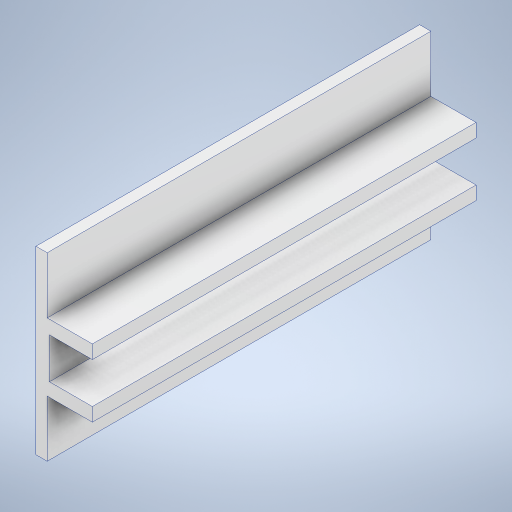
# Autodesk Inventor part: MainRails
Saved by Autodesk Inventor 2024 (Build 280153000, 153)
## iProperties
Created: 2023-08-20
Part Number: MainRails
Material: Aluminum 6061
Document SubType Name: Modeling
Designer: KirikDK
Mass: 4130.47 g
Surface Area: 1743.17 cm^2
Volume: 1529.8 cm^3
Density: 2.7 g/cm^3
Appearance: Aluminum - Flat
Author: KirikDK
Autodesk Inventor part; units mm, degrees
ref_plane "YZ Plane" through (0, 0, 0) normal (1, 0, 0) x (0, 1, 0)
ref_plane "XZ Plane" through (0, 0, 0) normal (0, 1, 0) x (-1, 0, 0)
ref_plane "XY Plane" through (0, 0, 0) normal (0, 0, 1) x (1, 0, 0)
sketch "Sketch1" plane through (0, 0, 0) normal (0, 1, 0) x (-1, 0, 0)
  line L0 (0, 279.3478) -> (-39.1304, 279.3478)
  line L1 (-39.1304, 279.3478) -> (-39.1304, -195.6522)
  line L2 (-39.1304, -195.6522) -> (0, -195.6522)
  line L3 (0, -195.6522) -> (0, 279.3478)
  line L4 (-39.1304, 279.3478) -> (-29.1304, 279.3478)
  line L5 (-29.1304, 254.3478) -> (-39.1304, 254.3478)
  line L6 (-39.1304, 254.3478) -> (-39.1304, 279.3478)
  line L7 (-39.1304, -195.6522) -> (-29.1304, -195.6522)
  line L8 (-29.1304, -170.6522) -> (-39.1304, -170.6522)
  line L9 (-39.1304, -170.6522) -> (-39.1304, -195.6522)
  point P0 (0, 0)
  point P1 (-39.1304, 254.3478)
  dimension "d0" = 475
  dimension "d4" = 25
  dimension "d5" = 25
  constraints: 20 end point, 4 parallel, 3 horizontal, 1 perpendicular
  measures "d0" distance of L2.end L0.start
  measures "d4" distance between parallel lines of L0 L5
  measures "d5" distance between parallel lines of L2 L8
extrude "Extrusion1" add sketch "Sketch1" along normal blind 160
sketch "Sketch2" plane through (0, 0, 279.3478) normal (0, 0, 1) x (1, 0, 0)
  line L0 (0, 160) -> (39.1304, 160) projected
  line L1 (0, 160) -> (39.1304, 160)
  line L2 (39.1304, 160) -> (39.1304, 0)
  line L3 (39.1304, 0) -> (0, 0)
  line L4 (0, 0) -> (0, 160)
  line L5 (39.1304, 160) -> (29.1304, 160)
  line L6 (29.1304, 160) -> (29.1304, 110)
  line L7 (29.1304, 110) -> (39.1304, 110)
  line L8 (39.1304, 110) -> (39.1304, 160)
  line L9 (39.1304, 0) -> (29.1304, 0)
  line L10 (29.1304, 0) -> (29.1304, 50)
  line L11 (29.1304, 50) -> (39.1304, 50)
  line L12 (39.1304, 50) -> (39.1304, 0)
  circle A0 centre (39.1304, 80) radius 18
  line L13 (31.1304, 75) -> (39.1304, 75)
  line L14 (39.1304, 75) -> (39.1304, 98)
  line L15 (39.1304, 98) -> (31.1304, 98)
  line L16 (31.1304, 98) -> (31.1304, 75)
  line L17 (31.1304, 75) -> (39.1304, 75)
  line L18 (39.1304, 75) -> (39.1304, 62)
  line L19 (39.1304, 62) -> (31.1304, 62)
  line L20 (31.1304, 62) -> (31.1304, 75)
  line L21 (39.1304, 0) -> (39.1304, 160) projected
  line L22 (0, 160) -> (19.1304, 160)
  line L23 (19.1304, 160) -> (19.1304, 0)
  line L24 (19.1304, 0) -> (0, 0)
  line L25 (0, 0) -> (0, 160)
  point P0 (0, 0)
  point P1 (34.1304, 110)
  point P2 (34.1304, 160)
  point P3 (39.1304, 50)
  point P4 (39.1304, 110)
  dimension "d6" = 10
  dimension "d7" = 50
  dimension "d8" = 50
  dimension "d9" = 8
  dimension "d10" = 36
  dimension "d11" = 80
  dimension "d12" = 80
  dimension "d15" = 20
  constraints: 48 end point, 12 parallel, 6 horizontal, 6 perpendicular, 4 point on line, 3 midpoint, 2 point on circle, 1 centre point, 3 other
  measures "d6" distance between parallel lines of L2 L10
  measures "d7" distance between parallel lines of L11 L3
  measures "d8" distance from line of L0 point (34.13, 110)
  measures "d9" distance between parallel lines of L2 L16
  measures "d10" diameter of A0
  measures "d11" distance from line of L3 point (39.13, 80)
  measures "d12" vertical distance of point (34.13, 160) point (39.13, 80)
  measures "d15" distance between parallel lines of L2 L23
extrude "Extrusion2" cut sketch "Sketch2" against normal up to surface (475 mm away) contours L0 L23 L3 L4 | L0 L2 L7 L6 | L10 L11 L2 L3 | L2 L13 L16 A0 | A0 L16 L15 | L2 A0 L20 L13 | L19 L20 A0
sketch "Sketch3" plane through (0, 160, 0) normal (0, 1, 0) x (1, 0, 0)
  line L0 (-18, 219) -> (160, 219)
  line L1 (160, 219) -> (160, 60.6522)
  line L2 (160, 60.6522) -> (-18, 60.6522)
  line L3 (-18, 60.6522) -> (-18, 219)
  line L4 (19.1304, -279.3478) -> (29.1304, -279.3478) projected
  point P0 (0, 0)
  dimension "d16" = 340
  constraints: 8 end point, 2 parallel, 1 horizontal, 1 perpendicular
  measures "d16" distance between parallel lines of L2 L4
extrude "Extrusion3" cut sketch "Sketch3" against normal blind 200
sketch "Sketch4" plane through (39.1304, 98, 279.3478) normal (1, 0, 0) x (0, 0, -1)
  line L0 (340, 0) -> (340, 12) projected
  line L1 (340, 12) -> (0, 12) projected
  line L2 (0, 0) -> (0, 12) projected
  line L3 (0, 0) -> (340, 0) projected
  line L4 (340, -48) -> (340, -36) projected
  line L5 (340, -36) -> (0, -36) projected
  line L6 (0, -48) -> (0, -36) projected
  line L7 (0, -48) -> (340, -48) projected
  point P0 (279.3478, -98)
extrude "Extrusion4" add sketch "Sketch4" along normal blind 30
body "Solid1"
